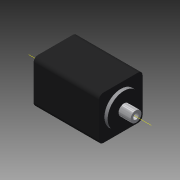
# Autodesk Inventor part: NEMA8
Saved by Autodesk Inventor 2015 (Build 190159000, 159)
## iProperties
Created: 2015-01-07
Part Number: NEMA8
Material: Generic
Document SubType Name: Modeling
Designer: ice
Density: 1 g/cm^3
Appearance: Default
Mass: 12.1989 g
Surface Area: 37.047 cm^2
Volume: 12.1989 cm^3
Author: ice
Autodesk Inventor part; units mm, degrees
ref_plane "YZ Plane" through (0, 0, 0) normal (1, 0, 0) x (0, 1, 0)
ref_plane "XZ Plane" through (0, 0, 0) normal (0, 1, 0) x (-1, 0, 0)
sketch "Sketch1" plane through (0, 0, 0) normal (0, 1, 0) x (-1, 0, 0)
  line L0 (0, 0) -> (0, -20)
  line L1 (0, -20) -> (30, -20)
  line L2 (30, -20) -> (30, 0)
  line L3 (30, 0) -> (0, 0)
  dimension "d0" = 20
  dimension "d1" = 30
  dimension "d2" = 20
  constraints: 8 end point, 2 perpendicular, 1 vertical
  measures "d0" distance of L0.start L0.end
  measures "d1" distance of L0.end L1.end
  measures "d2" distance of L1.end L2.end
extrude "Extrusion1" add sketch "Sketch1" along normal blind 20
sketch "Sketch2" plane through (0, 0, 0) normal (1, 0, 0) x (0, 0, -1)
  line L0 (0, 0) -> (20, 0) projected
  line L1 (10, 0) -> (10, 10)
  circle A0 centre (10, 10) radius 7.5
  dimension "d5" = 10
  dimension "d6" = 15
  constraints: 2 end point, 1 centre point, 1 coincident, 1 midpoint, 1 vertical
  measures "d5" distance of L1.start L1.end
  measures "d6" diameter of A0
extrude "Extrusion2" add sketch "Sketch2" along normal blind 1.5
sketch "Sketch3" plane through (1.5, 10, -10) normal (1, 0, 0) x (0, 0, -1)
  circle A0 centre (0, 0) radius 2.5
  point P0 (-10, -10)
  dimension "d9" = 5
  constraints: 1 centre point
  measures "d9" diameter of A0
extrude "Extrusion4" add sketch "Sketch3" along normal blind 5.5
sketch "Sketch4" plane through (-30, 0, -20) normal (-1, 0, 0) x (0, 0, 1)
  line L0 (20, 0) -> (0, 0) projected
  circle A0 centre (10, 10) radius 2.5 projected
  circle A1 centre (10, 10) radius 2.5
  dimension "d16" = 5
  constraints: 1 centre point, 1 coincident
  measures "d16" diameter of A1
extrude "Extrusion5" add sketch "Sketch4" along normal blind 7.5
sketch "Sketch5" plane through (-37.5, 10, -10) normal (-1, 0, 0) x (0, 0, 1)
  circle A0 centre (0, 0) radius 2.5
  point P0 (10, -10)
  dimension "d19" = 5
  constraints: 1 centre point
  measures "d19" diameter of A0
hole "Hole1" at (-37.5, 10, -10) direction (1, 0, 0) diameter 2.5 end through all
fillet "Fillet1" radius 2 4 edges at (-15, 20, -20) (-15, 20, 0) (-15, 0, -20) (-15, 0, 0)
ref_plane "Work Plane1" through (7, 10, -10) normal (1, 0, 0) x (0, 0, -1)
body "Solid1"
